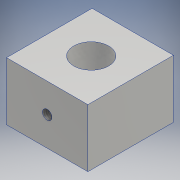
# Autodesk Inventor part: esbarro_carro
Saved by Autodesk Inventor 2018 (Build 220112000, 112)
## iProperties
Created: 2018-05-17
Part Number: esbarro_carro
Material: Alumínio 6061
Document SubType Name: Modeling
Designer: Usuario
Density: 2.7 g/cm^3
Appearance: Alumínio - Plano
Author: Usuario
Autodesk Inventor part; units mm, degrees
ref_plane "YZ Plane" through (0, 0, 0) normal (1, 0, 0) x (0, 1, 0)
ref_plane "XZ Plane" through (0, 0, 0) normal (0, 1, 0) x (-1, 0, 0)
ref_plane "XY Plane" through (0, 0, 0) normal (0, 0, 1) x (1, 0, 0)
sketch "Esboço1" plane through (0, 0, 0) normal (0, 0, 1) x (1, 0, 0)
  circle A0 centre (0, 0) radius 5.995 construction
  line L0 (13.9364, -15.0797) -> (-14.0636, -15.0797) construction
  line L1 (-14.0636, 14.3703) -> (13.9364, 14.3703)
  line L2 (13.9364, 14.3703) -> (13.9364, -15.0797)
  line L3 (13.9364, -15.0797) -> (-14.0636, -15.0797)
  line L4 (-14.0636, -15.0797) -> (-14.0636, 14.3703)
  circle A1 centre (0, 0) radius 6
  dimension "d0" = 12
  constraints: 8 end point, 2 parallel, 1 centre point, 1 coincident, 1 horizontal, 1 perpendicular
  measures "d0" diameter of A1
extrude "Extrusão1" add sketch "Esboço1" along normal blind 20
sketch "Esboço2" plane through (-14.0636, 14.3703, 0) normal (0, 1, 0) x (1, 0, 0)
  line L0 (28, 0) -> (28, -20) construction
  line L1 (0, 0) -> (0, -20) construction
  line L2 (28, -10) -> (0, -10) construction
  line L3 (14, -10) -> (14, 0) construction
  line L4 (14, -10) -> (5.5, -10) construction
  line L5 (14, -10) -> (22.5, -10) construction
  dimension "d7" = 10
  dimension "d8" = 8.5
  dimension "d9" = 8.5
  constraints: 8 end point, 3 midpoint, 2 point on line, 1 vertical
  measures "d7" distance of L3.start L3.end
  measures "d8" distance of L3.start L4.end
  measures "d9" distance of L3.start L5.end
hole "Furo1" at (8.4364, 14.3703, 10) at (-8.5636, 14.3703, 10) direction (0, -1, 0) diameter 3.242 depth 8 tip angle 118 thread size "M4x0.7" class "6H" standard "ANSI Metric M Profile"
sketch "Esboço3" plane through (-14.0636, -15.0797, 0) normal (0, -1, 0) x (1, 0, 0)
  line L0 (28, 20) -> (0, 20) projected
  line L1 (14, 20) -> (14, 0) construction
  circle A0 centre (14, 10) radius 2
  point P0 (14.0636, 0)
  dimension "d17" = 20
  dimension "d18" = 4
  constraints: 2 end point, 2 midpoint, 1 centre point, 1 vertical
  measures "d17" distance of L1.start L1.end
  measures "d18" diameter of A0
hole "Furo2" at (-0.0636, -15.0797, 10) direction (0, 1, 0) diameter 3.242 depth 10 tip angle 118 thread size "M4x0.7" class "6H" standard "ANSI Metric M Profile"
